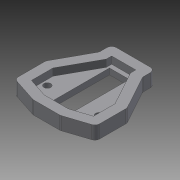
# Autodesk Inventor part: InkjetHolderV2
Saved by Autodesk Inventor 2015 (Build 190159000, 159)
## iProperties
Created: 2015-06-18
Part Number: InkjetHolderV2
Material: Generic
Document SubType Name: Modeling
Designer: Oliver
Density: 1 g/cm^3
Appearance: Default
Author: Oliver
Autodesk Inventor part; units mm, degrees
ref_plane "YZ Plane" through (0, 0, 0) normal (1, 0, 0) x (0, 1, 0)
ref_plane "XZ Plane" through (0, 0, 0) normal (0, 1, 0) x (-1, 0, 0)
ref_plane "XY Plane" through (0, 0, 0) normal (0, 0, 1) x (1, 0, 0)
sketch "Sketch1" plane through (0, 0, 0) normal (0, 0, 1) x (1, 0, 0)
  line L0 (-5, -2.5) -> (5, -2.5) construction
  line L1 (5, -2.5) -> (12.675, 0) construction
  line L2 (-5, -2.5) -> (-12.675, 0)
  line L3 (12.675, 0) -> (-12.675, 0) construction
  line L4 (12.675, 0) -> (12.675, 8.7) construction
  line L5 (-12.675, 0) -> (-12.675, 8.7)
  line L6 (-12.675, 8.7) -> (-4.75, 23.1)
  line L7 (-4.75, 23.1) -> (-4.75, 25.1)
  line L8 (-4.75, 25.1) -> (4.75, 25.1) construction
  line L9 (4.75, 25.1) -> (4.75, 23.1) construction
  line L10 (4.75, 23.1) -> (12.675, 8.7) construction
  line L11 (0, -8.44) -> (0, 31.04) projected
  line L12 (0, 25.1) -> (0, -2.5)
  circle A0 centre (-10.8, 4.25) radius 1.25
  line L13 (-10.8, 4.25) -> (0, 4.25) construction
  line L14 (-4.75, 25.1) -> (0, 25.1)
  line L15 (-5, -2.5) -> (0, -2.5)
  line L16 (-5.05, 23.1771) -> (-12.975, 8.7771)
  line L17 (-12.975, 8.7771) -> (-12.975, -0.2178)
  line L18 (-12.975, -0.2178) -> (-5.0476, -2.8)
  line L19 (-5.0476, -2.8) -> (0.3, -2.8) construction
  line L20 (0.3, -2.8) -> (0.3, 25.4) construction
  line L21 (0.3, 25.4) -> (-5.05, 25.4) construction
  line L22 (-5.05, 25.4) -> (-5.05, 23.1771)
  line L23 (0, -2.5) -> (0, -2.8)
  line L24 (0, 25.1) -> (0, 25.4)
  line L25 (0, -2.8) -> (-5.0476, -2.8)
  line L26 (0, 25.4) -> (-5.05, 25.4)
  point P0 (0, 0)
  point P1 (0, 0)
  dimension "d0" = 10
  dimension "d1" = 25.35
  dimension "d2" = 2.5
  dimension "d3" = 8.7
  dimension "d4" = 27.6
  dimension "d6" = 2
  dimension "d7" = 9.5
  dimension "d42" = 2.5
  dimension "d43" = 10.8
  dimension "d44" = 6.75
  dimension "d53" = 0.3
  constraints: 52 end point, 7 point on line, 4 equal length, 4 horizontal, 4 vertical, 3 collinear, 3 midpoint, 1 centre point, 1 coincident, 1 perpendicular, 6 other
  measures "d0" distance of L0.start L0.end
  measures "d1" distance of L1.end L2.end
  measures "d2" distance between parallel lines of L3 L0
  measures "d3" distance of L1.end L4.end
  measures "d4" distance between parallel lines of L0 L8
  measures "d6" distance of L8.end L9.end
  measures "d7" distance of L7.end L8.end
  measures "d42" diameter of A0
  measures "d43" distance of L13.start L13.end
  measures "d44" distance between parallel lines of L0 L13
  measures "d53" distance between parallel lines of L6 L16
sketch "Sketch8" plane through (0, 0, 0) normal (0, 0, 1) x (1, 0, 0)
  line L0 (-20, 30) -> (20, 30)
  line L1 (20, 30) -> (20, -10)
  line L2 (20, -10) -> (-20, -10)
  line L3 (-20, -10) -> (-20, 30)
  point P0 (0, 0)
  point P1 (0, -10)
  dimension "d45" = 40
  dimension "d46" = 10
  constraints: 8 end point, 2 parallel, 2 perpendicular, 1 horizontal, 1 midpoint, 1 vertical alignment
  measures "d45" distance of L1.end L2.end
  measures "d46" distance from line of L2 point (0, 0)
extrude "MainBlock" add sketch "Sketch8" against normal blind 5.5
extrude "CartridgeCutout" cut sketch "Sketch1" against normal blind 3
sketch "Sketch10" plane through (-10.8, 4.25, 0) normal (0, 0, 1) x (1, 0, 0)
  circle A0 centre (0, 0) radius 1.25 projected
  circle A1 centre (0, 0) radius 1.45
  point P0 (10.8, -4.25)
  dimension "d56" = 0.2
  constraints: 1 centre point
  measures "d56" radial gap between concentric circles of A0 A1
extrude "PinHole" cut sketch "Sketch10" against normal through all contours A0 | A1
mirror "Mirror3" about plane through (0, 25.4, 0) normal (-1, 0, 0) of "CartridgeCutout", "PinHole"
sketch "Sketch12" plane through (0, 0, -3) normal (0, 0, 1) x (1, 0, 0)
  circle A0 centre (10.8, 4.25) radius 1.45 projected
  circle A1 centre (-10.8, 4.25) radius 1.45 projected
  line L0 (5.05, 25.4) -> (-5.05, 25.4) projected
  line L1 (-5.05, 23.1771) -> (-5.05, 25.4) projected
  line L2 (-12.975, 8.7771) -> (-5.05, 23.1771) projected
  line L3 (-12.975, -0.2178) -> (-12.975, 8.7771) projected
  line L4 (-5.0476, -2.8) -> (-12.975, -0.2178) projected
  line L5 (5.0476, -2.8) -> (-5.0476, -2.8) projected
  line L6 (5.0476, -2.8) -> (12.975, -0.2178) projected
  line L7 (12.975, -0.2178) -> (12.975, 8.7771) projected
  line L8 (12.975, 8.7771) -> (5.05, 23.1771) projected
  line L9 (5.05, 23.1771) -> (5.05, 25.4) projected
  line L10 (-4.15, 23.6) -> (4.15, 23.6)
  line L11 (4.15, 23.6) -> (4.15, -1.4)
  line L12 (4.15, -1.4) -> (-4.15, -1.4)
  line L13 (-4.15, -1.4) -> (-4.15, 23.6)
  point P0 (0, 0)
  point P1 (0, -1.4)
  dimension "d59" = 8.3
  dimension "d60" = 25
  dimension "d61" = 1.4
  constraints: 8 end point, 2 parallel, 1 horizontal, 1 midpoint, 1 perpendicular, 1 vertical alignment
  measures "d59" distance of L11.end L12.end
  measures "d60" distance of L10.end L11.end
  measures "d61" distance from line of L12 point (0, 0)
extrude "Extrusion12" cut sketch "Sketch12" against normal through all contours L10 L11 L12 L13
sketch "Sketch13" plane through (0, 0, 0) normal (0, 0, 1) x (1, 0, 0)
  line L0 (-5.05, 25.4) -> (5.05, 25.4) projected
  line L1 (5.05, 25.4) -> (5.05, 23.1771) projected
  line L2 (5.05, 23.1771) -> (12.975, 8.7771) projected
  line L3 (12.975, 8.7771) -> (12.975, -0.2178) projected
  line L4 (12.975, -0.2178) -> (5.0476, -2.8) projected
  line L5 (5.0476, -2.8) -> (-5.0476, -2.8) projected
  line L6 (-5.0476, -2.8) -> (-12.975, -0.2178) projected
  line L7 (-12.975, -0.2178) -> (-12.975, 8.7771) projected
  line L8 (-12.975, 8.7771) -> (-5.05, 23.1771) projected
  line L9 (-5.05, 23.1771) -> (-5.05, 25.4) projected
  line L10 (-20, 30) -> (20, 30) projected
  line L11 (-20, -10) -> (-20, 30) projected
  line L12 (20, -10) -> (-20, -10) projected
  line L13 (20, 30) -> (20, -10) projected
  line L14 (-17, 9.8115) -> (-17, -3.1399)
  line L15 (-17, -3.1399) -> (-5.6866, -6.825)
  line L16 (-5.6866, -6.825) -> (5.6866, -6.825)
  line L17 (5.6866, -6.825) -> (17, -3.1399)
  line L18 (17, -3.1399) -> (17, 9.8115)
  line L19 (17, 9.8115) -> (9.075, 24.2115)
  line L20 (9.075, 24.2115) -> (9.075, 29.425)
  line L21 (9.075, 29.425) -> (-9.075, 29.425)
  line L22 (-9.075, 29.425) -> (-9.075, 24.2115)
  line L23 (-9.075, 24.2115) -> (-17, 9.8115)
  point P0 (0, 0)
  dimension "d65" = 4.025
  constraints: 20 end point, 9 other
  measures "d65" distance between parallel lines of L7 L14
extrude "Extrusion13" cut sketch "Sketch13" against normal through all contours L10 L13 L12 L11
fillet "Fillet2" radius 2 10 edges at (-9.075, 29.425, -2.75) (9.075, 29.425, -2.75) (9.075, 24.2115, -2.75) (17, 9.8115, -2.75) (17, -3.1399, -2.75) (5.6866, -6.825, -2.75) (-5.6866, -6.825, -2.75) (-17, -3.1399, -2.75) (-9.075, 24.2115, -2.75) (-17, 9.8115, -2.75)
body "Solid4"
